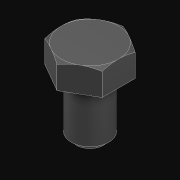
# Autodesk Inventor part: Screw Nylon Hex
Saved by Autodesk Inventor 2021 (Build 250183000, 183)
## iProperties
Created: 2021-07-20
Part Number: Screw Nylon Hex
Material: Black
Document SubType Name: Modeling
Designer: yuany
Density: 1.12 g/cm^3
Appearance: Nylon 6
Author: yuany
Autodesk Inventor part; units mm, degrees
ref_plane "YZ Plane" through (0, 0, 0) normal (1, 0, 0) x (0, 1, 0)
ref_plane "XZ Plane" through (0, 0, 0) normal (0, 1, 0) x (-1, 0, 0)
ref_plane "XY Plane" through (0, 0, 0) normal (0, 0, 1) x (1, 0, 0)
sketch "Sketch1" plane through (0, 0, 0) normal (0, 1, 0) x (-1, 0, 0)
  circle A0 centre (0, 0) radius 2.0828
  dimension "d0" = 4.1656
  constraints: 1 centre point, 1 coincident
  measures "d0" diameter of A0
extrude "Body" add sketch "Sketch1" along normal blind 6.35
sketch "Sketch2" plane through (0, 6.35, 0) normal (0, 1, 0) x (1, 0, 0)
  line L0 (-3.175, 1.8331) -> (0, 3.6662)
  line L1 (0, 3.6662) -> (3.175, 1.8331)
  line L2 (3.175, 1.8331) -> (3.175, -1.8331)
  line L3 (3.175, -1.8331) -> (0, -3.6662)
  line L4 (0, -3.6662) -> (-3.175, -1.8331)
  line L5 (-3.175, -1.8331) -> (-3.175, 1.8331)
  point P0 (0, 0)
  point P1 (0, 0)
  dimension "d3" = 6.35
  constraints: 12 end point, 1 coincident, 1 vertical, 13 other
  measures "d3" distance between parallel lines of L2 L5
extrude "Head" add sketch "Sketch2" along normal blind 2.794
sketch "Sketch3" plane through (0, 0, 0) normal (1, 0, 0) x (0, 1, 0)
  line L0 (8.8646, -3.6662) -> (9.144, -3.1822)
  line L1 (9.144, -3.1822) -> (9.144, -3.6662)
  line L2 (9.144, -3.6662) -> (8.8646, -3.6662)
  line L3 (6.35, -3.6662) -> (9.144, -3.6662) projected
  line L4 (9.144, -1.8331) -> (9.144, -3.6662) projected
  line L5 (-1.8288, 0) -> (10.9728, 0) projected
  point P0 (0, 0)
  dimension "d6" = 0.5588
  dimension "d7" = 60
  constraints: 6 end point, 2 collinear, 1 perpendicular, 1 vertical
  measures "d6" distance of L0.start L0.end
  measures "d7" angle of L2 L0
revolve "Head Chamfer" cut sketch "Sketch3" angle 360 about axis through (0, -10, 0) along (0, 1, 0)
sketch "Sketch4" plane through (0, 0, 0) normal (0, 0, 1) x (1, 0, 0)
  line L0 (-2.0828, 0) -> (-2.0828, 6.35) projected
  line L1 (-2.0828, 0.0762) -> (-2.0828, -0.6413)
  line L2 (-2.0828, -0.6413) -> (-2.6162, -0.3334)
  line L3 (-2.6162, -0.3334) -> (-2.6162, -0.2318)
  line L4 (-2.6162, -0.2318) -> (-2.0828, 0.0762)
  line L5 (2.0828, 0) -> (-2.0828, 0) projected
  point P0 (0, 0)
  dimension "d9" = 60
  dimension "d10" = 0.1016
  dimension "d11" = 0.0762
  dimension "d12" = 0.5334
  constraints: 8 end point, 1 collinear, 1 equal length, 1 parallel, 1 point on line
  measures "d9" angle of L4 L2
  measures "d10" distance of L2.end L3.end
  measures "d11" distance from line of L5 L1.start
  measures "d12" distance between parallel lines of L1 L3
feature "Thread" [suppressed]
sketch "Sketch5" plane through (0, 0, 0) normal (0, 0, 1) x (1, 0, 0)
  line L0 (0, 0) -> (-1.4986, 0)
  line L1 (-1.4986, 0) -> (-2.2461, 0.7475)
  line L2 (-2.2461, 0.7475) -> (-2.2461, -1.8711)
  line L3 (-2.2461, -1.8711) -> (-1.4986, -1.8711)
  line L4 (-1.4986, -1.8711) -> (-1.4986, 0)
  line L5 (-2.0828, 0) -> (-2.0828, 0) projected
  line L6 (0, -2.3949) -> (0, 1.2713) projected
  point P0 (0, 0)
  dimension "d21" = 1.4986
  dimension "d22" = 135
  dimension "d23" = 0
  dimension "d24" = 0
  constraints: 10 end point, 2 perpendicular, 1 horizontal, 1 vertical
  measures "d21" distance of L0.start L0.end
  measures "d22" angle of L1 L0
  measures "d23" distance of point (0, 0) L0.start
  measures "d24" distance between parallel lines of L5 L0
revolve "Tapered End" cut sketch "Sketch5" angle 360 about axis through (0, -10, 0) along (0, 1, 0)
body "Solid1"
